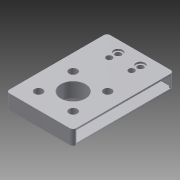
# Autodesk Inventor part: NEMA17-mount-extended-plastic
Saved by Autodesk Inventor 2015 (Build 190159000, 159)
## iProperties
Created: 2012-03-11
Part Number: NEMA17-mount-extended-plastic
Material: Generic
Document SubType Name: Modeling
Designer: Michael Green
Density: 1 g/cm^3
Appearance: Default
Author: Michael Green
Autodesk Inventor part; units mm, degrees
ref_plane "YZ Plane" through (0, 0, 0) normal (1, 0, 0) x (0, 1, 0)
ref_plane "XZ Plane" through (0, 0, 0) normal (0, 1, 0) x (-1, 0, 0)
ref_plane "XY Plane" through (0, 0, 0) normal (0, 0, 1) x (1, 0, 0)
sketch "base-drawing" plane through (0, 0, 0) normal (0, 0, 1) x (1, 0, 0)
  circle A0 centre (30, 30.15) radius 11.1
  line L0 (0, 0) -> (60, 0)
  circle A1 centre (45.5, 14.65) radius 1.7
  circle A2 centre (45.5, 45.65) radius 1.7
  circle A3 centre (14.5, 45.65) radius 1.7
  circle A4 centre (14.5, 14.65) radius 1.7
  line L1 (0, 0) -> (0, 90.5)
  line L2 (0, 90.5) -> (60, 90.5)
  line L3 (60, 90.5) -> (60, 0)
  circle A5 centre (40, 80.5) radius 2.65
  circle A6 centre (40, 72.5) radius 2.65
  circle A7 centre (20, 80.5) radius 2.65
  circle A8 centre (20, 72.5) radius 2.65
  line L4 (0, 0) -> (0, 45)
  line L5 (0, 60.5) -> (60, 60.5) construction
  dimension "d17" = 22.2
  dimension "d82" = 3.4
  dimension "d83" = 15.5
  dimension "d84" = 15.5
  dimension "d88" = 360
  dimension "d111" = 60
  dimension "d112" = 10
  dimension "d113" = 18
  dimension "d114" = 5.3
  dimension "d115" = 5.3
  dimension "d116" = 5.3
  dimension "d117" = 5.3
  dimension "d151" = 30
  dimension "d152" = 14.85
  dimension "d154" = 90.5
  constraints: 12 end point, 9 centre point, 4 coincident, 3 point on line, 2 horizontal alignment, 2 perpendicular, 1 horizontal, 1 parallel, 9 other
  measures "d17" diameter of A0
  measures "d82" diameter of A1
  measures "d83" horizontal distance of A1.centre A0.centre
  measures "d84" horizontal distance of A0.centre A1.centre
  measures "d111" distance of L0.end L0.start
  measures "d112" distance from line of point (20, 80.5) L2
  measures "d113" distance from line of L2 point (20, 72.5)
  measures "d114" diameter of A5
  measures "d115" diameter of A6
  measures "d116" diameter of A7
  measures "d117" diameter of A8
  measures "d151" distance between parallel lines of L5 L2
  measures "d152" distance from line of L5 A3.centre
  measures "d154" distance of L0.start L1.end
extrude "Extrusion4" add sketch "base-drawing" along normal blind 13
sketch "Sketch17" plane through (0, 0, 13) normal (0, 0, 1) x (1, 0, 0)
  circle A0 centre (14.5, 14.65) radius 1.7 projected
  circle A1 centre (14.5, 45.65) radius 1.7 projected
  circle A2 centre (45.5, 45.65) radius 1.7 projected
  circle A3 centre (45.5, 14.65) radius 1.7 projected
hole "Hole10" at (14.5, 45.65, 13) at (45.5, 45.65, 13) at (45.5, 14.65, 13) at (14.5, 14.65, 13) direction (0, 0, -1) diameter 7.3 depth 6.4
fillet "Fillet4" radius 3 4 edges at (0, 0, 6.5) (0, 90.5, 6.5) (60, 90.5, 6.5) (60, 0, 6.5)
shell "Shell6" thickness 1.5 removed faces 2 at (0, 59.3333, 8.6667) at (60, 31.1667, 4.3333)
sketch "Sketch20" plane through (0, 0, 13) normal (0, 0, 1) x (1, 0, 0)
  circle A0 centre (20, 80.5) radius 2.65 projected
  circle A1 centre (40, 80.5) radius 2.65 projected
  point P0 (0, 0)
hole "Hole13" at (40, 80.5, 13) at (20, 80.5, 13) direction (0, 0, -1) diameter 8 depth 1.5
sketch "Sketch21" plane through (0, 0, 0) normal (0, 0, -1) x (-1, 0, 0)
  circle A0 centre (-20, 80.5) radius 2.65 projected
  circle A1 centre (-40, 80.5) radius 2.65 projected
  point P0 (0, 0)
hole "Hole14" at (40, 80.5, 0) at (20, 80.5, 0) direction (0, 0, 1) diameter 8 depth 1.5
body "Solid4"
